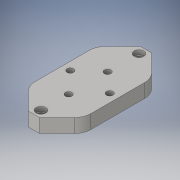
# Autodesk Inventor part: ROV Motor plate
Saved by Autodesk Inventor 2016 (Build 200138000, 138)
## iProperties
Created: 2017-03-09
Part Number: ROV Motor plate
Material: Generic
Document SubType Name: Modeling
Designer: Student
Density: 1 g/cm^3
Appearance: Default
Author: Student
Autodesk Inventor part; units mm, degrees
ref_plane "YZ Plane" through (0, 0, 0) normal (1, 0, 0) x (0, 1, 0)
ref_plane "XZ Plane" through (0, 0, 0) normal (0, 1, 0) x (-1, 0, 0)
ref_plane "XY Plane" through (0, 0, 0) normal (0, 0, 1) x (1, 0, 0)
sketch "Sketch1" plane through (0, 0, 0) normal (0, 1, 0) x (-1, 0, 0)
  line L0 (0, 0) -> (-25.4, 0)
  line L1 (-25.4, 0) -> (-25.4, -51.2064)
  line L2 (-25.4, -51.2064) -> (0, -51.2064)
  line L3 (0, -51.2064) -> (0, 0)
  dimension "d0" = 25.4
  dimension "d1" = 51.2064
  constraints: 8 end point, 2 parallel, 1 horizontal, 1 perpendicular
  measures "d0" distance of L2.end L1.end
  measures "d1" distance of L1.end L0.end
extrude "Extrusion1" add sketch "Sketch1" along normal blind 6.35
sketch "Sketch2" plane through (0, 6.35, 0) normal (0, 1, 0) x (1, 0, 0)
  line L0 (25.4, 51.2064) -> (0, 51.2064) projected
  line L1 (0, 0) -> (25.4, 0) projected
  line L2 (0, 51.2064) -> (0, 0) projected
  line L3 (25.4, 0) -> (25.4, 51.2064) projected
  point P0 (12.7, 48.0314)
  point P1 (12.7, 3.175)
  dimension "d6" = 3.175
  dimension "d8" = 12.7
  dimension "d10" = 12.7
  dimension "d37" = 3.175
  measures "d6" distance from line of L1 point (12.7, 3.175)
  measures "d8" distance from line of L2 point (12.7, 3.175)
  measures "d10" distance from line of L2 point (12.7, 48.031)
  measures "d37" distance from line of L0 point (12.7, 48.031)
hole "Hole1" at (12.7, 6.35, -48.0314) at (12.7, 6.35, -3.175) direction (0, -1, 0) diameter 3 end through all
sketch "Sketch3" plane through (0, 6.35, 0) normal (0, 1, 0) x (1, 0, 0)
  line L0 (25.4, 0) -> (25.4, 51.2064) projected
  line L1 (25.4, 51.2064) -> (0, 51.2064) projected
  line L2 (12.7, 51.2064) -> (12.7, -5.0328) construction
  point P0 (0, 0)
  point P1 (3.683, 25.6032)
  point P2 (21.717, 25.6032)
  point P3 (12.7, 33.654)
  point P4 (12.7, 15.8232)
  dimension "d26" = 25.6032
  dimension "d27" = 18.034
  dimension "d28" = 17.8308
  constraints: 2 end point, 2 point on line, 1 midpoint, 1 symmetric about line, 1 vertical
  measures "d26" distance from line of point (3.683, 25.603) L1
  measures "d27" distance of point (3.683, 25.603) point (21.717, 25.603)
  measures "d28" distance of point (12.7, 15.823) point (12.7, 33.654)
hole "Hole2" at (3.683, 6.35, -25.6032) at (21.717, 6.35, -25.6032) at (12.7, 6.35, -33.654) at (12.7, 6.35, -15.8232) direction (0, -1, 0) diameter 3 end through all
chamfer "Chamfer1" distance 10.16 angle 45 4 edges at (0, 3.175, -51.2064) (25.4, 3.175, -51.2064) (25.4, 3.175, 0) (0, 3.175, 0)
fillet "Fillet1" radius 7.62 4 edges at (0, 3.175, -41.0464) (0, 3.175, -10.16) (25.4, 3.175, -41.0464) (25.4, 3.175, -10.16)
sketch "Sketch5" plane through (0, 6.35, 0) normal (0, 1, 0) x (1, 0, 0)
  line L0 (0, 25.6032) -> (36.8771, 25.6032) construction
  circle A0 centre (12.7, 48.0314) radius 1.5 projected
  circle A1 centre (12.7, 48.0314) radius 2.2225
  circle A2 centre (12.7, 3.175) radius 1.5
  circle A3 centre (12.7, 3.175) radius 2.2225
  circle A4 centre (12.7, 15.8232) radius 1.5 projected
  circle A5 centre (12.7, 15.8232) radius 2.2225
  line L1 (15.24, 51.2064) -> (10.16, 51.2064) projected
  line L2 (12.7, 51.2064) -> (12.7, -4.6531) construction
  circle A6 centre (12.7, 35.3832) radius 1.5
  circle A7 centre (12.7, 35.3832) radius 2.2225
  point P0 (0, 0)
  dimension "d42" = 4.445
  dimension "d45" = 4.445
  constraints: 6 centre point, 4 coincident, 4 end point, 4 symmetric about line, 1 horizontal, 1 midpoint, 1 vertical, 4 other
  measures "d42" diameter of A1
  measures "d45" diameter of A5
extrude "Extrusion2" cut sketch "Sketch5" against normal blind 2.032 contours A1 | A3
body "Solid1"
